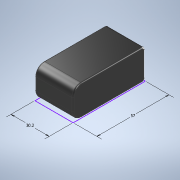
# Autodesk Inventor part: Lipo
Saved by Autodesk Inventor 2022 (Build 260153000, 153)
## iProperties
Created: 2021-10-08
Part Number: Lipo
Material: Generic
Document SubType Name: Modeling
Designer: tecware
Density: 1 g/cm^3
Appearance: Default
Author: tecware
Autodesk Inventor part; units mm, degrees
ref_plane "YZ Plane" through (0, 0, 0) normal (1, 0, 0) x (0, 1, 0)
ref_plane "XZ Plane" through (0, 0, 0) normal (0, 1, 0) x (-1, 0, 0)
ref_plane "XY Plane" through (0, 0, 0) normal (0, 0, 1) x (1, 0, 0)
sketch "Sketch1" plane through (0, 0, 0) normal (0, 1, 0) x (-1, 0, 0)
  line L0 (15.1, -28.5) -> (-15.1, -28.5)
  line L1 (-15.1, -28.5) -> (-15.1, 28.5)
  line L2 (-15.1, 28.5) -> (15.1, 28.5)
  line L3 (15.1, 28.5) -> (15.1, -28.5)
  dimension "d0" = 30.2
  dimension "d1" = 57
  constraints: 8 end point, 2 parallel, 1 horizontal, 1 perpendicular
  measures "d0" distance of L1.end L2.end
  measures "d1" distance of L0.end L1.end
extrude "Extrusion1" add sketch "Sketch1" along normal blind 23.7
fillet "Fillet1" radius 2 2 edges at (0, 23.7, -28.5) (0, 0, -28.5)
fillet "Fillet2" radius 7 2 edges at (0, 23.7, 28.5) (0, 0, 28.5)
fillet "Fillet3" radius 1 16 edges at (15.1, 23.7, -2.5) (15.1, 23.1142, -27.9142) (15.1, 11.85, -28.5) (15.1, 0.5858, -27.9142) (15.1, 0, -2.5) (15.1, 2.0503, 26.4497) (15.1, 11.85, 28.5) (15.1, 21.6497, 26.4497) (-15.1, 21.6497, 26.4497) (-15.1, 11.85, 28.5) (-15.1, 2.0503, 26.4497) (-15.1, 0, -2.5) (-15.1, 0.5858, -27.9142) (-15.1, 11.85, -28.5) (-15.1, 23.1142, -27.9142) (-15.1, 23.7, -2.5)
body "Solid1"
